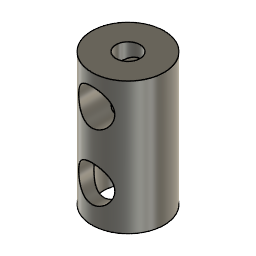
軸接合装置 v1 (Autodesk Fusion 360 design; units mm, degrees)
Autodesk Fusion 360 part; units mm, degrees
sketch "スケッチ1" plane through (0, 0, 0) normal (0, 0, 1) x (1, 0, 0)
  circle A0 centre (0, 0) radius 1
  circle A1 centre (0, 0) radius 3
  constraint coincident A0.centre A1.centre
  constraint concentric A0 A1
extrude "押し出し1" add sketch "スケッチ1" along normal blind 5
sketch "スケッチ2" plane through (0, 0, 0) normal (0, 0, -1) x (1, 0, 0)
  circle A0 centre (0, 0) radius 1
  circle A1 centre (0, 0) radius 3
  circle A2 centre (0, 0) radius 2
  constraint concentric A0 A2
extrude "押し出し2" add sketch "スケッチ2" along normal blind 6 contours A1
ref_plane "作業平面1" through (0, 0, -0.5) normal (0, 1, 0) x (0, 0, 1)
sketch "スケッチ3" plane through (0, 0, 0) normal (0, 1, 0) x (1, 0, 0)
  circle A0 centre (0, -2.5) radius 1.5
  circle A1 centre (0, 3) radius 1.5
extrude "押し出し3" cut sketch "スケッチ3" along normal mid plane 6
